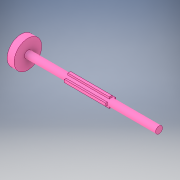
# Autodesk Inventor part: ShaftForWormGear
Saved by Autodesk Inventor 2019.3 (Build 233278000, 278)
## iProperties
Created: 2019-01-06
Part Number: ShaftForWormGear
Material: PBT Plastic
Document SubType Name: Modeling
Designer: steele
Density: 1.31 g/cm^3
Appearance: Pink
Author: steele
Autodesk Inventor part; units mm, degrees
ref_plane "YZ Plane" through (0, 0, 0) normal (1, 0, 0) x (0, 1, 0)
ref_plane "XZ Plane" through (0, 0, 0) normal (0, 1, 0) x (-1, 0, 0)
sketch "Sketch2" plane through (0, 0, 0) normal (1, 0, 0) x (0, 1, 0)
  circle A0 centre (0, 0) radius 3.175
  dimension "d0" = 6.35
  constraints: 1 centre point, 1 coincident
  measures "d0" diameter of A0
extrude "Extrusion1" add sketch "Sketch2" along normal mid plane 127
sketch "Sketch3" plane through (-63.5, 0, 0) normal (-1, 0, 0) x (0, 0, 1)
  circle A0 centre (0, 0) radius 12.7
  dimension "d3" = 25.4
  constraints: 1 centre point, 1 coincident
  measures "d3" diameter of A0
extrude "Extrusion2" add sketch "Sketch3" against normal blind 6.35
sketch "Sketch4" plane through (-57.15, 0, 0) normal (1, 0, 0) x (0, 0, -1)
  line L0 (0, 4.572) -> (1.27, 4.572)
  line L1 (1.27, 4.572) -> (1.27, 2.9099)
  circle A0 centre (0, 0) radius 3.175 projected
  line L2 (0, -17.78) -> (0, 17.78) projected
  line L3 (0, 4.572) -> (-1.27, 4.572)
  line L4 (-1.27, 4.572) -> (-1.27, 2.9099)
  line L5 (-4.572, 0) -> (-4.572, -1.27)
  line L6 (-4.572, 0) -> (-4.572, 1.27)
  line L7 (-4.572, 1.27) -> (-2.9099, 1.27)
  line L8 (-4.572, -1.27) -> (-2.9099, -1.27)
  line L9 (0, -4.572) -> (1.27, -4.572)
  line L10 (0, -4.572) -> (-1.27, -4.572)
  line L11 (-1.27, -4.572) -> (-1.27, -2.9099)
  line L12 (1.27, -4.572) -> (1.27, -2.9099)
  line L13 (4.572, 0) -> (4.572, 1.27)
  line L14 (4.572, 0) -> (4.572, -1.27)
  line L15 (4.572, -1.27) -> (2.9099, -1.27)
  line L16 (4.572, 1.27) -> (2.9099, 1.27)
  arc A1 (1.27, 2.9099) -> (-1.27, 2.9099) centre (0, 0) ccw
  arc A2 (2.9099, -1.27) -> (2.9099, 1.27) centre (0, 0) ccw
  arc A3 (-2.9099, 1.27) -> (-2.9099, -1.27) centre (0, 0) ccw
  arc A4 (-1.27, -2.9099) -> (1.27, -2.9099) centre (0, 0) ccw
  dimension "d7" = 1.27
  dimension "d10" = 360
  dimension "d15" = 1.397
  constraints: 32 end point, 8 point on circle, 4 centre point, 2 symmetric about line, 1 coincident, 1 horizontal, 1 perpendicular, 39 other
  measures "d7" distance between parallel lines of L1 L2
  measures "d15" distance edge to line of A1 L3
extrude "Extrusion3" add sketch "Sketch4" along normal blind 76.2 contours L0 L1 A0 L2 | L2 A0 L4 L3 | L2 L10 L11 A0 | A0 L12 L9 L2 | L16 L13 L14 L15 A0 | A0 L8 L5 L6 L7
ref_plane "Work Plane1" through (-19.05, 0, 0) normal (1, 0, 0) x (0, 0, -1)
sketch "Sketch5" plane through (-19.05, 0, 0) normal (1, 0, 0) x (0, 0, -1)
  circle A0 centre (0, 0) radius 3.175
  circle A1 centre (0, 0) radius 5.4209
  constraints: 2 centre point, 2 coincident
extrude "Extrusion4" cut sketch "Sketch5" against normal blind 38.1
body "Solid1"
